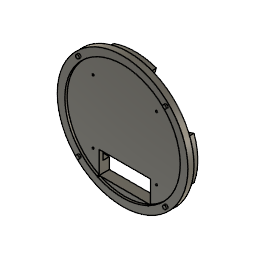
Cover_Plate (Autodesk Fusion 360 design; units mm, degrees)
Autodesk Fusion 360 part; units mm, degrees
sketch "Sketch1" plane through (0, 0, 0) normal (0, 1, 0) x (1, 0, 0)
  circle A0 centre (0, 0) radius 102
  dimension "d1" = 204
  constraint coincident A0.centre origin
  measures "d1" diameter of A0
extrude "Extrude1" add sketch "Sketch1" along normal blind 6
sketch "Sketch2" plane through (0, 0, 0) normal (0, -1, 0) x (1, 0, 0)
  circle A0 centre (0, 0) radius 102
  circle A1 centre (0, 0) radius 102
  circle A2 centre (0, 0) radius 90
  dimension "d4" = 204
  dimension "d5" = 180
  constraint concentric A0 A1
  constraint concentric A1 A2
  measures "d4" diameter of A1
  measures "d5" diameter of A2
extrude "Extrude2" add sketch "Sketch2" along normal blind 3.5
sketch "Sketch3" plane through (0, -3.5, 0) normal (0, -1, 0) x (1, 0, 0)
  circle A0 centre (0, 0) radius 90
  circle A1 centre (0, 0) radius 102
  circle A2 centre (0, 0) radius 96 construction
  line L0 (0, 0) -> (-67.8823, 67.8823) construction
  line L1 (0, 0) -> (96, 0) construction
  line L2 (0, 0) -> (67.8823, 67.8823) construction
  line L3 (0, 0) -> (96, 0) construction
  line L4 (0, 0) -> (-67.8823, -67.8823) construction
  line L5 (0, 0) -> (96, 0) construction
  line L6 (0, 0) -> (67.8823, -67.8823) construction
  line L7 (0, 0) -> (96, 0) construction
  circle A3 centre (-67.8823, 67.8823) radius 2.925
  circle A4 centre (67.8823, 67.8823) radius 2.925
  circle A5 centre (-67.8823, -67.8823) radius 2.925
  circle A6 centre (67.8823, -67.8823) radius 2.925
  dimension "d8" = 192
  dimension "d9" = 135
  dimension "d10" = 45
  dimension "d11" = 135
  dimension "d12" = 45
  dimension "d13" = 5.85
  dimension "d14" = 5.85
  dimension "d15" = 5.85
  dimension "d16" = 5.85
  constraint concentric A0 A2
  constraint horizontal L1
  constraint coincident A0.centre A1.centre
  constraint horizontal L3
  constraint horizontal L5
  constraint horizontal L7
  constraint coincident L0.end A3.centre
  constraint coincident L2.end A4.centre
  constraint coincident L4.end A5.centre
  constraint coincident L6.end A6.centre
  measures "d8" diameter of A2
  measures "d9" angle of L0 L1
  measures "d10" angle of L2 L3
  measures "d11" angle of L4 L5
  measures "d12" angle of L6 L7
  measures "d13" diameter of A3
  measures "d14" diameter of A4
  measures "d15" diameter of A5
  measures "d16" diameter of A6
extrude "Extrude3" add sketch "Sketch3" along normal blind 2.5 contours A3 | A4 | A5 | A6
sketch "Sketch4" plane through (0, 6, 0) normal (0, 1, 0) x (-1, 0, 0)
  circle A0 centre (0, 0) radius 102
  line L0 (0, 0) -> (0, -64) construction
  line L1 (40, -81.5) -> (-40, -81.5)
  line L2 (-40, -81.5) -> (-40, -46.5)
  line L3 (-40, -46.5) -> (40, -46.5)
  line L4 (40, -46.5) -> (40, -81.5)
  line L5 (40, -81.5) -> (-40, -46.5) construction
  line L6 (-40, -81.5) -> (40, -46.5) construction
  point P0 (0, -64)
  dimension "d19" = 64
  dimension "d20" = 80
  dimension "d21" = 35
  constraint coincident A0.centre L0.start
  constraint vertical L0
  constraint horizontal L1
  constraint perpendicular L1 L2
  constraint parallel L1 L3
  constraint parallel L2 L4
  constraint coincident L5 P0
  constraint coincident L6 P0
  constraint coincident P0 L0.end
  measures "d19" distance of A0.centre P0
  measures "d20" distance of L2.end L3.end
  measures "d21" distance of L1.end L2.end
extrude "Extrude4" cut sketch "Sketch4" against normal blind 20 contours L1 L2 L3 L4
sketch "Sketch5" plane through (0, 6, 0) normal (0, 1, 0) x (-1, 0, 0)
  line L0 (-40, -81.5) -> (-40, -46.5)
  line L1 (-40, -46.5) -> (40, -46.5)
  line L2 (40, -46.5) -> (40, -81.5)
  line L3 (40, -81.5) -> (-40, -81.5)
  circle A0 centre (0, 0) radius 102
  line L4 (40, 0) -> (-40, 0)
  arc A1 (40, 0) -> (-40, 0) centre (0, 0) ccw
  circle A2 centre (0, 0) radius 70 construction
  line L5 (0, 0) -> (49.4975, -49.4975) construction
  line L6 (0, 0) -> (70, 0) construction
  line L7 (0, 0) -> (49.4975, 49.4975) construction
  line L8 (0, 0) -> (70, 0) construction
  line L9 (0, 0) -> (-49.4975, -49.4975) construction
  line L10 (0, 0) -> (70, 0) construction
  line L11 (0, 0) -> (-49.4975, 49.4975) construction
  line L12 (0, 0) -> (70, 0) construction
  line L13 (0, 0) -> (98, 0) construction
  line L14 (0, 0) -> (98, 0) construction
  line L15 (0, 0) -> (98, 0) construction
  line L16 (-82.693, 30.0978) -> (-92.0899, 33.518)
  line L17 (0, 0) -> (98, 0) construction
  line L18 (30.0978, 82.693) -> (33.518, 92.0899)
  line L19 (0, 0) -> (98, 0) construction
  line L20 (-30.0978, 82.693) -> (-33.518, 92.0899)
  line L21 (0, 0) -> (98, 0) construction
  line L22 (82.693, -30.0978) -> (92.0899, -33.518)
  line L23 (82.693, 30.0978) -> (92.0899, 33.518)
  line L24 (-82.693, -30.0978) -> (-92.0899, -33.518)
  line L25 (60.1951, -64.1915) -> (74.0503, -64.1915)
  line L26 (-60.1951, -64.1915) -> (-74.0503, -64.1915)
  arc A3 (-74.0503, -64.1915) -> (74.0503, -64.1915) centre (0, 0) ccw
  arc A4 (-82.693, 30.0978) -> (-82.693, -30.0978) centre (0, 0) ccw
  arc A5 (-92.0899, 33.518) -> (-92.0899, -33.518) centre (0, 0) ccw
  arc A6 (92.0899, -33.518) -> (92.0899, 33.518) centre (0, 0) ccw
  arc A7 (33.518, 92.0899) -> (-33.518, 92.0899) centre (0, 0) ccw
  arc A8 (82.693, -30.0978) -> (82.693, 30.0978) centre (0, 0) ccw
  arc A9 (30.0978, 82.693) -> (-30.0978, 82.693) centre (0, 0) ccw
  line L27 (-60.1951, -64.1915) -> (-40, -64.1915)
  line L28 (40, -64.1915) -> (60.1951, -64.1915)
  circle A10 centre (49.4975, -49.4975) radius 1.5
  circle A11 centre (49.4975, -49.4975) radius 3
  circle A12 centre (-49.4975, -49.4975) radius 1.5
  circle A13 centre (-49.4975, -49.4975) radius 3
  circle A14 centre (49.4975, 49.4975) radius 1.5
  circle A15 centre (49.4975, 49.4975) radius 3
  circle A16 centre (-49.4975, 49.4975) radius 1.5
  circle A17 centre (-49.4975, 49.4975) radius 3
  dimension "d24" = 176
  dimension "d25" = 196
  dimension "d26" = 80
  dimension "d27" = 140
  dimension "d28" = 45
  dimension "d29" = 45
  dimension "d30" = 135
  dimension "d31" = 135
  dimension "d35" = 160
  dimension "d36" = 70
  dimension "d37" = 110
  dimension "d38" = 3
  dimension "d39" = 6
  dimension "d40" = 3
  dimension "d41" = 6
  dimension "d42" = 3
  dimension "d43" = 6
  dimension "d44" = 3
  dimension "d45" = 6
  constraint concentric A0 A3
  constraint concentric A0 A1
  constraint horizontal L4
  constraint perpendicular L0 L27
  constraint concentric A0 A2
  constraint horizontal L6
  constraint coincident A0.centre A1.centre
  constraint horizontal L8
  constraint horizontal L10
  constraint horizontal L12
  constraint horizontal L13
  constraint horizontal L14
  constraint horizontal L15
  constraint horizontal L17
  constraint horizontal L19
  constraint horizontal L21
  constraint parallel L25 L28
  constraint parallel L26 L27
  constraint concentric A3 A5
  constraint concentric A4 A9
  constraint concentric A5 A7
  constraint concentric A6 A7
  constraint concentric A8 A9
  constraint collinear L27 L28
  constraint coincident L0 L27.end
  constraint coincident L2 L28.start
  constraint coincident L5.end A10.centre
  constraint concentric A10 A11
  constraint coincident L9.end A12.centre
  constraint concentric A12 A13
  constraint coincident L7.end A14.centre
  constraint concentric A14 A15
  constraint coincident L11.end A16.centre
  measures "d24" diameter of A8
  measures "d25" diameter of A6
  measures "d26" diameter of A1
  measures "d27" diameter of A2
  measures "d28" angle of L5 L6
  measures "d29" angle of L7 L8
  measures "d30" angle of L9 L10
  measures "d31" angle of L11 L12
  measures "d35" angle of L16 L17
  measures "d36" angle of L18 L19
  measures "d37" angle of L20 L21
  measures "d38" diameter of A10
  measures "d39" diameter of A11
  measures "d40" diameter of A12
  measures "d41" diameter of A13
  measures "d42" diameter of A14
  measures "d43" diameter of A15
  measures "d44" diameter of A16
  measures "d45" diameter of A17
extrude "Extrude5" cut sketch "Sketch5" against normal blind 20 contours A10 | A12 | A14 | A16
extrude "Extrude6" cut sketch "Sketch5" against normal blind 4 contours A11 | A13 | A15 | A17
extrude "Extrude7" add sketch "Sketch5" along normal blind 10 contours L0 L2 L3 L25 L26 A3 L27 L28 | L4 A1 | L16 L24 A4 A5 | L18 L20 A7 A9 | L22 L23 A6 A8
sketch "Sketch6" plane through (0, 16, 0) normal (0, 1, 0) x (-1, 0, 0)
  arc A0 (40, 0) -> (-40, 0) centre (0, 0) ccw
  line L0 (-40, 0) -> (40, 0)
  circle A1 centre (0, 0) radius 93 construction
  circle A2 centre (0, 0) radius 20 construction
  line L1 (0, 0) -> (0, 20) construction
  line L2 (0, 0) -> (91.5871, -16.1493) construction
  line L3 (0, 0) -> (93, 0) construction
  line L4 (0, 0) -> (91.5871, 16.1493) construction
  line L5 (0, 0) -> (93, 0) construction
  line L6 (0, 0) -> (-91.5871, -16.1493) construction
  line L7 (0, 0) -> (93, 0) construction
  line L8 (0, 0) -> (-91.5871, 16.1493) construction
  line L9 (0, 0) -> (93, 0) construction
  line L10 (0, 0) -> (16.1493, 91.5871) construction
  line L11 (0, 0) -> (93, 0) construction
  line L12 (0, 0) -> (-16.1493, 91.5871) construction
  line L13 (0, 0) -> (93, 0) construction
  line L14 (0, 0) -> (0, -93) construction
  line L15 (0, 0) -> (-53.3426, -76.1811) construction
  line L16 (0, 0) -> (53.3426, -76.1811) construction
  circle A3 centre (0, -93) radius 3
  circle A4 centre (-53.3426, -76.1811) radius 3
  circle A5 centre (53.3426, -76.1811) radius 3
  circle A6 centre (91.5871, -16.1493) radius 3
  circle A7 centre (91.5871, 16.1493) radius 3
  circle A8 centre (-91.5871, -16.1493) radius 3
  circle A9 centre (-91.5871, 16.1493) radius 3
  circle A10 centre (-16.1493, 91.5871) radius 3
  circle A11 centre (16.1493, 91.5871) radius 3
  circle A12 centre (0, 20) radius 3
  dimension "d52" = 186
  dimension "d53" = 40
  dimension "d54" = 10
  dimension "d55" = 10
  dimension "d56" = 170
  dimension "d57" = 170
  dimension "d58" = 80
  dimension "d59" = 100
  dimension "d60" = 145
  dimension "d61" = 6
  dimension "d62" = 6
  dimension "d63" = 6
  dimension "d64" = 6
  dimension "d65" = 6
  dimension "d66" = 6
  dimension "d67" = 6
  dimension "d68" = 6
  dimension "d69" = 6
  dimension "d70" = 6
  constraint concentric A0 A1
  constraint concentric A0 A2
  constraint coincident A0.centre A1.centre
  constraint coincident A2 L1.end
  constraint perpendicular L0 L1
  constraint horizontal L3
  constraint horizontal L5
  constraint horizontal L7
  constraint horizontal L9
  constraint horizontal L11
  constraint horizontal L13
  constraint coincident A1 L14.end
  constraint vertical L14
  constraint symmetric A0.centre L14 A1.centre
  constraint symmetric L14 L15.end L16.end
  constraint coincident L14.end A3.centre
  constraint coincident L15.end A4.centre
  constraint coincident L16.end A5.centre
  constraint coincident L2.end A6.centre
  constraint coincident L4.end A7.centre
  constraint coincident L6.end A8.centre
  constraint coincident L8.end A9.centre
  constraint coincident L12.end A10.centre
  constraint coincident L10.end A11.centre
  constraint coincident L1.end A12.centre
  measures "d52" diameter of A1
  measures "d53" diameter of A2
  measures "d54" angle of L2 L3
  measures "d55" angle of L4 L5
  measures "d56" angle of L6 L7
  measures "d57" angle of L8 L9
  measures "d58" angle of L10 L11
  measures "d59" angle of L12 L13
  measures "d60" angle of L14 L15
  measures "d61" diameter of A3
  measures "d62" diameter of A4
  measures "d63" diameter of A5
  measures "d64" diameter of A6
  measures "d65" diameter of A7
  measures "d66" diameter of A8
  measures "d67" diameter of A9
  measures "d68" diameter of A10
  measures "d69" diameter of A11
  measures "d70" diameter of A12
extrude "Extrude8" cut sketch "Sketch6" against normal blind 3.2 contours A3 | A4 | A5 | A6 | A7 | A8 | A9 | A10 | A11 | A12
